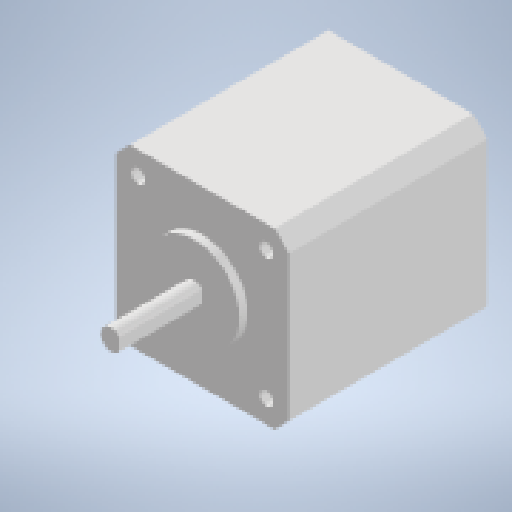
# Autodesk Inventor part: motor_x
Saved by Autodesk Inventor 2024 (Build 280153000, 153)
## iProperties
Created: 2026-02-04
Part Number: motor_x
Material: Generic
Document SubType Name: Modeling
Designer: SEMEN
Density: 1 g/cm^3
Appearance: Default
Author: SEMEN
Autodesk Inventor part; units mm, degrees
ref_plane "YZ Plane" through (0, 0, 0) normal (1, 0, 0) x (0, 1, 0)
ref_plane "XZ Plane" through (0, 0, 0) normal (0, 1, 0) x (-1, 0, 0)
ref_plane "XY Plane" through (0, 0, 0) normal (0, 0, 1) x (1, 0, 0)
sketch "Sketch1" plane through (0, 0, 0) normal (0, 0, 1) x (1, 0, 0)
  line L0 (21, -21) -> (-21, -21)
  line L1 (-21, -21) -> (-21, 21)
  line L2 (-21, 21) -> (21, 21)
  line L3 (21, 21) -> (21, -21)
  line L4 (21, -21) -> (-21, 21) construction
  line L5 (-21, -21) -> (21, 21) construction
  circle A0 centre (0, 0) radius 11
  circle A1 centre (0, 0) radius 2.5
  line L6 (2, 1.5) -> (2, -1.5)
  line L7 (0, 21) -> (0, -21) construction
  line L8 (-21, 0) -> (21, 0) construction
  point P0 (-15.5, 15.5)
  point P1 (15.5, 15.5)
  point P2 (15.5, -15.5)
  point P3 (-15.5, -15.5)
  dimension "d0" = 42
  dimension "d1" = 42
  dimension "d2" = 22
  dimension "d3" = 5
  dimension "d4" = 2
  dimension "d5" = 31
  constraints: 18 end point, 6 midpoint, 4 point on line, 3 symmetric about line, 2 centre point, 2 coincident, 2 parallel, 2 point on circle, 1 horizontal, 1 perpendicular, 1 vertical
  measures "d0" distance of L1.end L2.end
  measures "d1" distance of L0.end L1.end
  measures "d2" diameter of A0
  measures "d3" diameter of A1
  measures "d4" distance from line of point (0, 0) L6
  measures "d5" distance of point (15.5, 15.5) point (-15.5, 15.5)
extrude "Extrusion1" add sketch "Sketch1" against normal blind 48 contours L0 L1 L2 L3 | A0 | A1 L6 | L6 A1
extrude "Extrusion2" add sketch "Sketch1" along normal blind 2 contours A0 | A1 L6 | L6 A1
extrude "Extrusion3" add sketch "Sketch1" along normal blind 22 contours L6 A1 picked at (0.2258, 0.7583)
hole "Hole1" at (-15.5, -15.5, 0) at (-15.5, 15.5, 0) at (15.5, 15.5, 0) at (15.5, -15.5, 0) direction (0, 0, -1) diameter 3.4 depth 4.5 clearance for "Countersunk Head GOST 12876-67" size "M3" standard "GOST"
chamfer "Chamfer1" distance 3.5 angle 45 4 edges at (-21, -21, -24) (-21, 21, -24) (21, -21, -24) (21, 21, -24)
body "Solid1"
